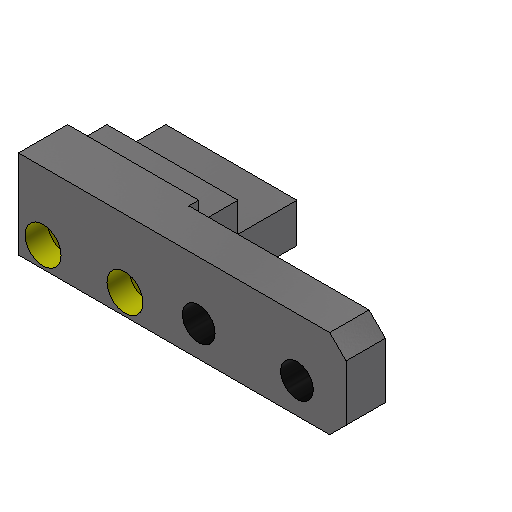
# Autodesk Inventor part: TL20240901-10320CV-013
Saved by Autodesk Inventor 2022.5 (Build 265521000, 521)
## iProperties
Category: FOLLOWER UNIT ASSY
Company: 현대 트랜시스
Created: 2023-05-03
Part Number: TL20240901-10320CV-013
Checked By: 김형민
Engr Approved By: 김형민
User Status: 1/1 x6
Material: SS400
Description: 0
Document SubType Name: Modeling
Mfg Approved By: 호상태
Designer: 박성규
Stock Number: 013
Density: 7.85 g/cm^3
Appearance: Plating Zinc White
Project: MEa-PJT 2LINE
DETAIL: Coveryor Assembly
M/C TITLE: CJ 제일제당 협동로봇 포장시스탬 PILOT 장비
PARTS NAME: Bracket
SPECIFICATION: TA20221101-CV200000-015
DocNumber: 221118_Standard_v1
Folder: .\
VDS_Category: 엔지니어링
Detail Description: Processed products
Title: BLOCK
Subject: MEa차종 시트조립2라인
Author: 박성규
Revision Number: A
Autodesk Inventor part; units mm, degrees
ref_plane "YZ Plane" through (0, 0, 0) normal (1, 0, 0) x (0, 1, 0)
ref_plane "XZ Plane" through (0, 0, 0) normal (0, 1, 0) x (-1, 0, 0)
ref_plane "XY Plane" through (0, 0, 0) normal (0, 0, 1) x (1, 0, 0)
sketch "스케치9" plane through (0, 0, 0) normal (0, 0, 1) x (1, 0, 0)
  line L0 (50, -13.5) -> (-50, -13.5)
  line L1 (-50, -13.5) -> (-50, 13.5)
  line L2 (-50, 13.5) -> (50, 13.5)
  line L3 (50, 13.5) -> (50, -13.5)
  line L4 (50, -13.5) -> (-50, 13.5) construction
  line L5 (-50, -13.5) -> (50, 13.5) construction
  point P0 (0, 0)
  dimension "d40" = 27
  dimension "d41" = 100
  constraints: 12 end point, 2 midpoint, 2 parallel, 1 horizontal, 1 perpendicular
  measures "d40" distance of L0.end L1.end
  measures "d41" distance of L0.start L0.end
extrude "돌출4" add sketch "스케치9" along normal blind 45
sketch "스케치10" plane through (50, -13.5, 0) normal (1, 0, 0) x (0, 0, -1)
  line L0 (0, 27) -> (0, 0) construction
  line L1 (0, 27) -> (-18, 27)
  line L2 (-18, 27) -> (-18, 12)
  line L3 (-18, 12) -> (0, 12)
  line L4 (0, 12) -> (0, 27)
  point P0 (0, 13.5)
  dimension "d44" = 18
  dimension "d51" = 15
  constraints: 8 end point, 2 parallel, 1 horizontal, 1 perpendicular
  measures "d44" distance of L2.end L3.end
  measures "d51" distance of L1.end L2.end
extrude "돌출5" cut sketch "스케치10" against normal through all
sketch "스케치11" plane through (50, -13.5, 45) normal (1, 0, 0) x (0, 0, -1)
  line L0 (27, 27) -> (0, 27) construction
  line L1 (45, 0) -> (45, 12) construction
  line L2 (45, 0) -> (12, 0)
  line L3 (12, 0) -> (12, 27)
  line L4 (12, 27) -> (45, 27)
  line L5 (45, 27) -> (45, 0)
  point P0 (45, 13.5)
  dimension "d48" = 33
  constraints: 8 end point, 2 parallel, 1 horizontal, 1 perpendicular, 1 point on line
  measures "d48" distance between parallel lines of L1 L3
extrude "돌출6" cut sketch "스케치11" against normal blind 60
sketch "스케치12" plane through (0, 0, 45) normal (0, 0, 1) x (1, 0, 0)
  line L0 (-50, -13.5) -> (50, -13.5) construction
  line L1 (50, -13.5) -> (50, 13.5) construction
  point P0 (0, 0)
  point P1 (35, -4.15)
  point P2 (5, -4.15)
  dimension "d52" = 9.35
  dimension "d53" = 15
  dimension "d54" = 30
  constraints: 1 horizontal alignment
  measures "d52" distance from line of L0 point (35, -4.15)
  measures "d53" distance from line of point (35, -4.15) L1
  measures "d54" distance of point (5, -4.15) point (35, -4.15)
hole "구멍3" at (35, -4.15, 45) at (5, -4.15, 45) direction (0, 0, -1) diameter 10 end through all
sketch "스케치13" plane through (0, 0, 45) normal (0, 0, 1) x (1, 0, 0)
  line L0 (-50, 13.5) -> (-50, -13.5) construction
  line L1 (-50, -13.5) -> (50, -13.5) construction
  point P0 (0, 0)
  point P1 (-17.5, -7.15)
  point P2 (-42.5, -7.15)
  dimension "d62" = 7.5
  dimension "d63" = 25
  dimension "d64" = 6.35
  constraints: 1 horizontal alignment
  measures "d62" distance from line of L0 point (-42.5, -7.15)
  measures "d63" distance of point (-17.5, -7.15) point (-42.5, -7.15)
  measures "d64" distance from line of L1 point (-42.5, -7.15)
hole "구멍4" at (-17.5, -7.15, 45) at (-42.5, -7.15, 45) direction (0, 0, -1) diameter 6.6 end through all counterbore diameter 11 counterbore depth 6.8 clearance for "Socket Head Cap Screw ISO 4762" size "M6" standard "ISO"
chamfer "모따기1" distance 5 angle 45 2 edges at (50, 13.5, 39) (50, -13.5, 39)
sketch "스케치14" plane through (-50, -13.5, 45) normal (-1, 0, 0) x (0, 0, 1)
  line L0 (-27, 27) -> (-27, 12) projected
  line L1 (-27, 27) -> (-15, 27)
  line L2 (-15, 27) -> (-15, 21)
  line L3 (-15, 21) -> (-27, 21)
  line L4 (-27, 21) -> (-27, 27)
  point P0 (-45, 13.5)
  dimension "d78" = 12
  dimension "d79" = 6
  constraints: 8 end point, 2 parallel, 1 horizontal, 1 perpendicular
  measures "d78" distance of L1.end L0.start
  measures "d79" distance of L3.end L0.start
extrude "돌출7" cut sketch "스케치14" against normal through all
